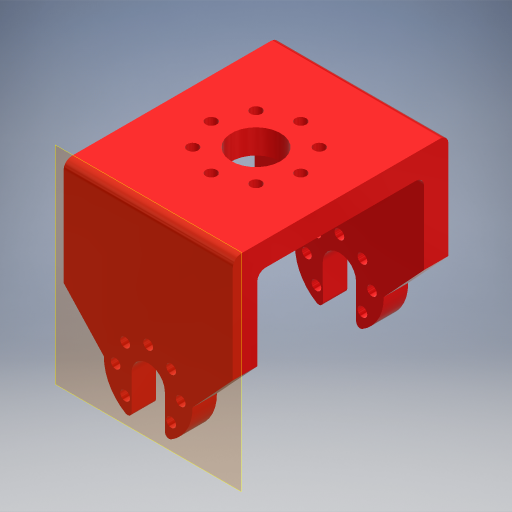
# Autodesk Inventor part: shoulder_ver2_new
Saved by Autodesk Inventor 2024 (Build 280153000, 153)
## iProperties
Created: 2024-09-08
Part Number: shoulder_ver2_new
Material: PMMA 플라스틱
Document SubType Name: Modeling
Designer: msi
Density: 1.188 g/cm^3
Appearance: 매끄러움 - 빨간색
Author: msi
Autodesk Inventor part; units mm, degrees
ref_plane "YZ Plane" through (0, 0, 0) normal (1, 0, 0) x (0, 1, 0)
ref_plane "XZ Plane" through (0, 0, 0) normal (0, 1, 0) x (-1, 0, 0)
ref_plane "XY Plane" through (0, 0, 0) normal (0, 0, 1) x (1, 0, 0)
ref_plane "작업 평면1" through (0, 0, 0) normal (0, 0, 1) x (1, 0, 0)
sketch "스케치1" plane through (0, 0, 0) normal (0, 0, 1) x (1, 0, 0)
  arc A0 (5.05, 17.3607) -> (6.05, 18.3607) centre (6.05, 17.3607) ccw projected
  line L0 (5.05, 17.3607) -> (-5.05, 17.3607) projected
  arc A1 (-6.05, 18.3607) -> (-5.05, 17.3607) centre (-6.05, 17.3607) ccw projected
  line L1 (-6.05, 18.3607) -> (-6.05, 23.4607) projected
  line L2 (-6.05, 23.4607) -> (-20.8, 23.4607) projected
  line L3 (-20.8, 23.4607) -> (-20.8, -2.5393) projected
  line L4 (-20.8, -2.5393) -> (-10.8995, -13.2319) projected
  arc A2 (-10.8995, -13.2319) -> (-5.5649, -22.7117) centre (0, -13.3393) ccw projected
  arc A3 (-5.5649, -22.7117) -> (-4.0544, -21.8465) centre (-5.0543, -21.8519) ccw projected
  line L5 (-4.0544, -21.8465) -> (-4.0998, -13.3833) projected
  arc A4 (4.1, -13.3393) -> (-4.0998, -13.3833) centre (0, -13.3393) ccw projected
  line L6 (4.1, -13.3393) -> (4.1, -21.8246) projected
  arc A5 (4.1, -21.8246) -> (5.6152, -22.6817) centre (5.1, -21.8246) ccw projected
  arc A6 (5.6152, -22.6817) -> (10.8995, -13.2319) centre (0, -13.3393) ccw projected
  line L7 (10.8995, -13.2319) -> (20.8, -2.5393) projected
  line L8 (20.8, -2.5393) -> (20.8, 23.4607) projected
  line L9 (20.8, 23.4607) -> (6.05, 23.4607) projected
  line L10 (6.05, 23.4607) -> (6.05, 18.3607) projected
  circle A7 centre (5.6569, -18.9962) radius 1.2 projected
  circle A8 centre (5.6569, -7.6825) radius 1.2 projected
  circle A9 centre (-5.6569, -7.6825) radius 1.2 projected
  circle A10 centre (0, -5.3393) radius 1.2 projected
  circle A11 centre (8, -13.3393) radius 1.2 projected
  circle A12 centre (-15.8, 20.4107) radius 1.35 projected
  circle A13 centre (15.8, 20.4107) radius 1.35 projected
  circle A14 centre (-8, -13.3393) radius 1.2 projected
  circle A15 centre (-5.6569, -18.9962) radius 1.2 projected
  line L11 (-20.8, 23.4607) -> (20.8, 23.4607)
  line L12 (20.8, 23.4607) -> (20.8, -2.5393)
  line L13 (20.8, -2.5393) -> (-20.8, -2.5393)
  line L14 (-20.8, -2.5393) -> (-20.8, 23.4607)
  circle A16 centre (0, -13.3393) radius 4.1
  circle A17 centre (0, -13.3393) radius 10.9
  circle A18 centre (0, -5.3393) radius 1.2
  circle A19 centre (-5.6569, -7.6825) radius 1.2
  circle A20 centre (-8, -13.3393) radius 1.2
  circle A21 centre (-5.6569, -18.9962) radius 1.2
  circle A22 centre (0, -21.3393) radius 1.2
  circle A23 centre (5.6569, -18.9962) radius 1.2
  circle A24 centre (8, -13.3393) radius 1.2
  circle A25 centre (5.6569, -7.6825) radius 1.2
  line L15 (-20.8, -2.5393) -> (-10.8995, -13.2319)
  line L16 (10.8995, -13.2319) -> (20.8, -2.5393)
  point P0 (0, 0)
  point P1 (-1.4731, -2.5393)
  point P2 (1.4731, -2.5393)
  dimension "d2" = 360
  constraints: 12 end point, 9 centre point, 3 coincident, 2 concentric, 2 parallel, 1 horizontal, 1 horizontal alignment, 1 perpendicular, 19 other
extrude "돌출1" add sketch "스케치1" against normal blind 6 contours L0 A1 L1 L11 L10 A0 | A0 L10 L9 L8 L13 A17 L3 L2 L1 A1 L0 | L7 A17 L13 | A6 A5 L6 A4 L5 A3 A2 A17 L13 | L13 A17 L4 | A12 | A13
sketch "스케치2" plane through (0, 0, -6) normal (0, 0, -1) x (-1, 0, 0)
  circle A0 centre (-5.6569, -18.9962) radius 1.2 projected
  circle A1 centre (-5.6569, -7.6825) radius 1.2 projected
  circle A2 centre (5.6569, -7.6825) radius 1.2 projected
  circle A3 centre (0, -5.3393) radius 1.2 projected
  circle A4 centre (-8, -13.3393) radius 1.2 projected
  circle A5 centre (15.8, 20.4107) radius 1.35 projected
  circle A6 centre (-15.8, 20.4107) radius 1.35 projected
  circle A7 centre (8, -13.3393) radius 1.2 projected
  circle A8 centre (5.6569, -18.9962) radius 1.2 projected
  arc A9 (-6.05, 18.3607) -> (-5.05, 17.3607) centre (-6.05, 17.3607) ccw projected
  line L0 (-6.05, 18.3607) -> (-6.05, 23.4607) projected
  line L1 (-20.8, 23.4607) -> (-6.05, 23.4607) projected
  line L2 (-20.8, -2.5393) -> (-20.8, 23.4607) projected
  line L3 (-10.8995, -13.2319) -> (-20.8, -2.5393) projected
  arc A10 (-10.8995, -13.2319) -> (-5.6152, -22.6817) centre (0, -13.3393) ccw projected
  arc A11 (-5.6152, -22.6817) -> (-4.1, -21.8246) centre (-5.1, -21.8246) ccw projected
  line L4 (-4.1, -13.3393) -> (-4.1, -21.8246) projected
  arc A12 (4.0998, -13.3833) -> (-4.1, -13.3393) centre (0, -13.3393) ccw projected
  line L5 (4.0544, -21.8465) -> (4.0998, -13.3833) projected
  arc A13 (4.0544, -21.8465) -> (5.5649, -22.7117) centre (5.0543, -21.8519) ccw projected
  arc A14 (5.5649, -22.7117) -> (10.8995, -13.2319) centre (0, -13.3393) ccw projected
  line L6 (20.8, -2.5393) -> (10.8995, -13.2319) projected
  line L7 (20.8, 23.4607) -> (20.8, -2.5393) projected
  line L8 (6.05, 23.4607) -> (20.8, 23.4607) projected
  line L9 (6.05, 23.4607) -> (6.05, 18.3607) projected
  arc A15 (5.05, 17.3607) -> (6.05, 18.3607) centre (6.05, 17.3607) ccw projected
  line L10 (5.05, 17.3607) -> (-5.05, 17.3607) projected
  line L11 (-20.8, 23.4607) -> (20.8, 23.4607)
  line L12 (20.8, 23.4607) -> (20.8, 17.4607)
  line L13 (20.8, 17.4607) -> (-20.8, 17.4607)
  line L14 (-20.8, 17.4607) -> (-20.8, 23.4607)
  point P0 (0, 0)
  dimension "d6" = 6
  constraints: 8 end point, 2 parallel, 1 horizontal, 1 perpendicular, 1 point on line
  measures "d6" distance of L11.end L12.end
extrude "돌출2" add sketch "스케치2" along normal blind 20.5 contours A5 | A6 | L0 L11 L9 A15 L13 A9 | A9 L13 L2 L1 L0 | A15 L9 L8 L7 L13
sketch "스케치3" plane through (-20.8, 23.4607, 0) normal (0, 1, 0) x (1, 0, 0)
  line L0 (39.2, 41.4) -> (34, 41.4) projected
  line L1 (34, 41.4) -> (34, 43.6) projected
  line L2 (34, 43.6) -> (39.2, 43.6) projected
  line L3 (39.2, 43.6) -> (39.2, 41.4) projected
  line L4 (2.4, 11.6) -> (7.6, 11.6) projected
  line L5 (7.6, 11.6) -> (7.6, 9.4) projected
  line L6 (7.6, 9.4) -> (2.4, 9.4) projected
  line L7 (2.4, 9.4) -> (2.4, 11.6) projected
  line L8 (39.2, 11.6) -> (39.2, 9.4) projected
  line L9 (39.2, 9.4) -> (34, 9.4) projected
  line L10 (34, 9.4) -> (34, 11.6) projected
  line L11 (34, 11.6) -> (39.2, 11.6) projected
  line L12 (7.6, 41.4) -> (2.4, 41.4) projected
  line L13 (2.4, 41.4) -> (2.4, 43.6) projected
  line L14 (2.4, 43.6) -> (7.6, 43.6) projected
  line L15 (7.6, 43.6) -> (7.6, 41.4) projected
  line L16 (14.8, 47) -> (-0.2, 47) projected
  line L17 (-0.2, 47) -> (-0.2, 6) projected
  line L18 (-0.2, 6) -> (14.8, 6) projected
  line L19 (14.8, 0) -> (14.8, 6) projected
  line L20 (26.8, 0) -> (14.8, 0) projected
  line L21 (26.8, 0) -> (26.8, 6) projected
  line L22 (26.8, 6) -> (41.8, 6) projected
  line L23 (41.8, 6) -> (41.8, 47) projected
  line L24 (41.8, 47) -> (26.8, 47) projected
  line L25 (26.8, 53) -> (26.8, 47) projected
  line L26 (14.8, 53) -> (26.8, 53) projected
  line L27 (14.8, 53) -> (14.8, 47) projected
  circle A0 centre (20.8, 26.5) radius 6 projected
  circle A1 centre (20.8, 37.5) radius 1.6 projected
  circle A2 centre (13.0218, 34.2782) radius 1.6 projected
  circle A3 centre (9.8, 26.5) radius 1.6 projected
  circle A4 centre (13.0218, 18.7218) radius 1.6 projected
  circle A5 centre (20.8, 15.5) radius 1.6 projected
  circle A6 centre (28.5782, 18.7218) radius 1.6 projected
  circle A7 centre (31.8, 26.5) radius 1.6 projected
  circle A8 centre (28.5782, 34.2782) radius 1.6 projected
  circle A9 centre (20.8, 26.5) radius 6
  circle A10 centre (13.0218, 18.7218) radius 1.35
  circle A11 centre (20.8, 15.5) radius 1.35
  circle A12 centre (28.5782, 18.7218) radius 1.35
  circle A13 centre (31.8, 26.5) radius 1.35
  circle A14 centre (28.5782, 34.2782) radius 1.35
  circle A15 centre (20.8, 37.5) radius 1.35
  circle A16 centre (13.0218, 34.2782) radius 1.35
  circle A17 centre (9.8, 26.5) radius 1.35
  point P0 (20.8, 0)
  dimension "d9" = 2.7
  dimension "d12" = 360
  constraints: 9 centre point, 2 coincident, 1 concentric, 17 other
  measures "d9" diameter of A10
extrude "돌출3" cut sketch "스케치3" against normal blind 20.5 contours A0 | A10 | A11 | A12 | A13 | A17
mirror "미러1" about plane through (0, 20.4607, -26.5) normal (0, 0, -1)
fillet "모깎기1" radius 2 4 edges at (0, 17.4607, -6) (0, 17.4607, -47) (0, 23.4607, -53) (0, 23.4607, 0)
sketch "스케치4" plane through (0, 0, 0) normal (0, 0, 1) x (1, 0, 0)
  line L0 (1.4731, -2.5393) -> (-1.4731, -2.5393) projected
  arc A0 (1.4731, -2.5393) -> (-1.4731, -2.5393) centre (0, -13.3393) ccw projected
  line L1 (-1.6142, -2.1682) -> (1.6887, -2.1682)
  line L2 (1.6887, -2.1682) -> (1.6887, -3.0074)
  line L3 (1.6887, -3.0074) -> (-1.6142, -3.0074)
  line L4 (-1.6142, -3.0074) -> (-1.6142, -2.1682)
  point P0 (0, 0)
  constraints: 8 end point, 2 parallel, 1 horizontal, 1 perpendicular
extrude "돌출4" add sketch "스케치4" against normal blind 6 contours L0 A0 | L1 L2 L3 L4
sketch "스케치5" plane through (4.1, -21.8246, -53) normal (0, 0, -1) x (-1, 0, 0)
  line L0 (2.2483, 20.1118) -> (6.3529, 20.1118)
  line L1 (6.3529, 20.1118) -> (6.3529, 18.3836)
  line L2 (6.3529, 18.3836) -> (2.2483, 18.3836)
  line L3 (2.2483, 18.3836) -> (2.2483, 20.1118)
  point P0 (4.1, 21.8246)
  constraints: 8 end point, 2 parallel, 1 horizontal, 1 perpendicular
extrude "돌출5" add sketch "스케치5" against normal blind 6
